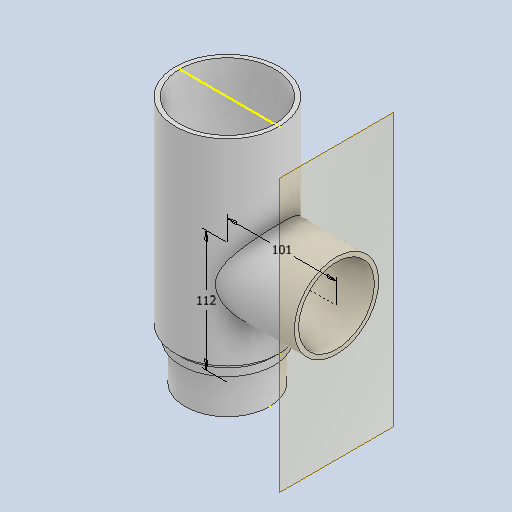
# Autodesk Inventor part: 7_Cuerpo
Saved by Autodesk Inventor 2024.3 (Build 283343000, 343)
## iProperties
Created: 2024-04-27
Part Number: 7_Cuerpo
Material: Genérico
Document SubType Name: Modeling
Designer: Cosmic Dinodog
Density: 1 g/cm^3
Appearance: Valor por defecto
Author: Cosmic Dinodog
Autodesk Inventor part; units mm, degrees
ref_plane "XZ Plane" through (0, 0, 0) normal (0, 1, 0) x (-1, 0, 0)
ref_plane "XY Plane" through (0, 0, 0) normal (0, 0, 1) x (1, 0, 0)
sketch "Boceto1" plane through (0, 0, 0) normal (0, 0, 1) x (1, 0, 0)
  line L0 (0, 0) -> (39, 0) construction
  line L1 (39, 0) -> (39, 35)
  line L2 (39, 35) -> (43, 35)
  line L3 (43, 35) -> (43, 42)
  arc A0 (48, 47) -> (43, 42) centre (48, 42) ccw
  line L4 (48, 47) -> (48, 229)
  line L5 (0, 0) -> (0, 229) construction
  line L6 (48, 229) -> (44, 229)
  line L7 (0, 112) -> (48, 112) construction
  line L8 (48, 112) -> (48, 77) construction
  line L9 (48, 77) -> (48, 56) construction
  line L10 (44, 229) -> (44, 56)
  line L11 (44, 56) -> (40, 56)
  line L12 (40, 56) -> (40, 65)
  line L13 (40, 65) -> (35, 60)
  line L14 (39, 0) -> (35, 0)
  line L15 (35, 0) -> (35, 60)
  dimension "d0" = 39
  dimension "d1" = 35
  dimension "d2" = 4
  dimension "d7" = 5
  dimension "d9" = 229
  dimension "d10" = 12
  dimension "d11" = 5
  dimension "d12" = 182
  dimension "d13" = 4
  dimension "d14" = 117
  dimension "d15" = 35
  dimension "d16" = 21
  dimension "d17" = 4
  dimension "d18" = 9
  dimension "d19" = 45
  dimension "d20" = 4
  dimension "d21" = 173
  constraints: 32 end point, 5 perpendicular, 5 point on line, 3 vertical, 2 horizontal, 2 parallel, 2 point on circle, 1 centre point, 1 tangent
  measures "d0" distance of L0.start L0.end
  measures "d1" distance of L0.end L1.end
  measures "d2" distance of L1.end L2.end
  measures "d7" radius of A0
  measures "d9" distance of L0.start L5.end
  measures "d10" vertical distance of L2.end L4.start
  measures "d11" horizontal distance of L4.start L2.end
  measures "d12" distance of L4.start L4.end
  measures "d13" distance of L4.end L6.end
  measures "d14" distance from line of L7 L5.end
  measures "d15" distance of L7.end L8.end
  measures "d16" distance of L8.end L9.end
  measures "d17" distance of L10.end L11.end
  measures "d18" distance of L11.end L12.end
  measures "d19" angle of L13 L12
  measures "d20" distance of L0.end L14.end
  measures "d21" distance between parallel lines of L11 L6
revolve "Revolución1" add sketch "Boceto1" angle 360 about axis through (0, 0, 0) along (0, 1, 0)
sketch "Boceto2" plane through (0, 0, 0) normal (0, 0, 1) x (1, 0, 0)
  line L0 (48, 229) -> (-48, 229) projected
  line L1 (48, 47) -> (-48, 47) projected
  line L2 (39, 35) -> (-39, 35) projected
  line L3 (39, 0) -> (-39, 0) projected
  line L4 (0, 0) -> (0, 112) construction
  line L5 (0, 112) -> (101, 112) construction
  dimension "d23" = 112
  dimension "d24" = 101
  constraints: 4 end point, 1 perpendicular, 1 vertical
  measures "d23" distance of L4.start L4.end
  measures "d24" distance of L4.end L5.end
ref_plane "Plano de trabajo1" through (101, 112, 0) normal (1, 0, 0) x (0, 1, 0)
sketch "Boceto3" plane through (101, 112, 0) normal (1, 0, 0) x (0, 1, 0)
  circle A0 centre (0, 0) radius 39
  point P0 (-112, 0)
  dimension "d25" = 78
  dimension "d26" = 112
  constraints: 1 centre point
  measures "d25" diameter of A0
  measures "d26" distance of point (-112, 0) A0.centre
extrude "Extrusión1" add sketch "Boceto3" against normal up to surface
sketch "Boceto4" plane through (101, 112, 0) normal (1, 0, 0) x (0, 0, -1)
  circle A0 centre (0, 0) radius 35
  circle A1 centre (0, 0) radius 39 projected
  point P0 (0, -112)
  dimension "d29" = 70
  dimension "d30" = 4
  constraints: 1 centre point
  measures "d29" diameter of A0
  measures "d30" radial gap between concentric circles of A1 A0
extrude "Extrusión2" cut sketch "Boceto4" against normal up to surface contours A0
